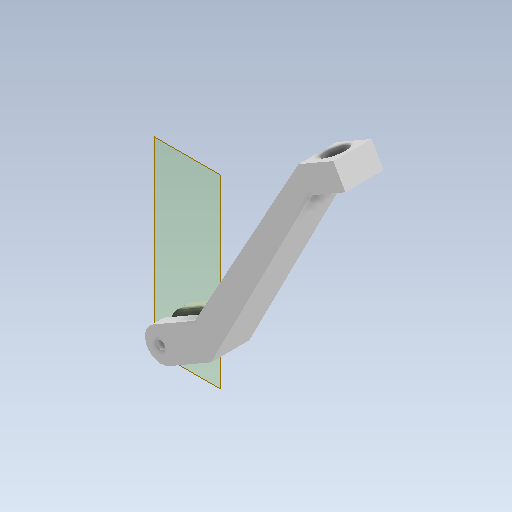
# Autodesk Inventor part: Union_dedo_base
Saved by Autodesk Inventor 2020 (Build 240168000, 168)
## iProperties
Created: 2021-07-22
Part Number: Union_dedo_base
Material: Generic
Document SubType Name: Modeling
Designer: chalo
Density: 1 g/cm^3
Appearance: Default
Author: chalo
Autodesk Inventor part; units mm, degrees
ref_plane "YZ Plane" through (0, 0, 0) normal (1, 0, 0) x (0, 1, 0)
ref_plane "XZ Plane" through (0, 0, 0) normal (0, 1, 0) x (-1, 0, 0)
ref_plane "XY Plane" through (0, 0, 0) normal (0, 0, 1) x (1, 0, 0)
sketch "Sketch1" plane through (0, 0, 0) normal (0, 0, 1) x (1, 0, 0)
  circle A0 centre (0, -7.23) radius 0.5 projected
  circle A1 centre (0, -7.23) radius 2
  point P0 (0, 0)
  dimension "d0" = 4
  constraints: 1 centre point, 1 coincident
  measures "d0" diameter of A1
extrude "Extrusion1" add sketch "Sketch1" along normal blind 1.5
sketch "Sketch2" plane through (0, -7.23, 1.5) normal (0, 0, 1) x (1, 0, 0)
  circle A0 centre (0, 0) radius 2 projected
  circle A1 centre (0, 0) radius 0.5 projected
  circle A2 centre (0, 0) radius 2 projected
  line L0 (1, -1.7321) -> (6.1962, 1.2679)
  line L1 (-1, 1.7321) -> (4.1962, 4.7321)
  line L2 (22.8311, 17.6353) -> (-6.9601, 0.4353) construction
  circle A3 centre (0, 0) radius 2 projected
  line L3 (4.1962, 4.7321) -> (17.0361, 27.9727)
  line L4 (6.1962, 1.2679) -> (18.5361, 25.3746)
  line L5 (4.1962, 4.7321) -> (6.1962, 1.2679) construction
  line L6 (18.5361, 25.3746) -> (17.0361, 27.9727)
  line L7 (15.8361, 30.0512) -> (18.5361, 25.3746) construction
  point P0 (0, 7.23)
  point P1 (-1, 1.7321)
  point P2 (1, -1.7321)
  dimension "d4" = 6
  dimension "d13" = 3
  constraints: 13 end point, 2 parallel, 2 perpendicular, 2 point on circle, 2 point on line, 2 tangent
  measures "d4" distance of L0.start L0.end
  measures "d13" distance of L4.end L3.end
extrude "Extrusion2" add sketch "Sketch2" against normal blind 1.5 contours A0 L1 L3 L6 L4 L0
ref_plane "Work Plane1" through (0, 0, -1.75) normal (0, 0, -1) x (-1, 0, 0)
sketch "Sketch3" plane through (0, 0, -1.75) normal (0, 0, -1) x (-1, 0, 0)
  line L0 (1, -5.4979) -> (-4.1962, -2.4979) projected
  line L1 (-4.1962, -2.4979) -> (-17.0361, 20.7427) projected
  line L2 (-17.0361, 20.7427) -> (-18.5361, 18.1446) projected
  line L3 (-18.5361, 18.1446) -> (-6.1962, -5.9621) projected
  line L4 (-6.1962, -5.9621) -> (-1, -8.9621) projected
  arc A0 (-1, -8.9621) -> (1, -5.4979) centre (0, -7.23) ccw projected
  circle A1 centre (0, -7.23) radius 0.5 projected
  point P0 (0, 0)
extrude "Extrusion3" add sketch "Sketch3" along normal blind 1.5
sketch "Sketch4" plane through (0, 0, 0) normal (0, 0, -1) x (-1, 0, 0)
  line L0 (-17.0361, 20.7427) -> (-18.5361, 18.1446) projected
  line L1 (-18.5361, 18.1446) -> (-6.1962, -5.9621) projected
  line L2 (-6.1962, -5.9621) -> (-1, -8.9621) projected
  arc A0 (-1, -8.9621) -> (1, -5.4979) centre (0, -7.23) ccw projected
  line L3 (1, -5.4979) -> (-4.1962, -2.4979) projected
  line L4 (-4.1962, -2.4979) -> (-17.0361, 20.7427) projected
  circle A1 centre (0, -7.23) radius 0.5 projected
  line L5 (1, -5.4979) -> (-4.1962, -2.4979) projected
  line L6 (-4.1962, -2.4979) -> (-6.1962, -5.9621)
  point P0 (0, 0)
  constraints: 2 end point
extrude "Extrusion4" add sketch "Sketch4" along normal up to next contours L4 L6 L1 L0
sketch "Sketch5" plane through (18.5361, 18.1446, 1.5) normal (0.8660254, 0.5, 0) x (0, 0, -1)
  line L0 (0, 0) -> (0, 3) projected
  line L1 (0, 0) -> (4.75, 0) projected
  line L2 (4.75, 3) -> (4.75, 0) projected
  line L3 (0, 3) -> (4.75, 3) projected
  point P0 (1.5, -6.4457)
extrude "Extrusion5" add sketch "Sketch5" along normal blind 5
sketch "Sketch6" plane through (18.5361, 18.1446, -3.25) normal (0.5, -0.8660254, 0) x (0.8660254, 0.5, 0)
  line L0 (0, 4.75) -> (0, 0) projected
  line L1 (0, 0) -> (5, 0) projected
  line L2 (5, 4.75) -> (5, 0) projected
  line L3 (0, 4.75) -> (5, 4.75) projected
  circle A0 centre (2.5, 2.375) radius 1.5
  point P0 (-25.125, 3.25)
  point P1 (0, 2.375)
  point P2 (2.5, 0)
  dimension "d14" = 3
  constraints: 2 midpoint, 1 centre point, 1 horizontal alignment, 1 vertical alignment
  measures "d14" diameter of A0
extrude "Extrusion6" cut sketch "Sketch6" against normal up to next contours A0
body "Solid1"
